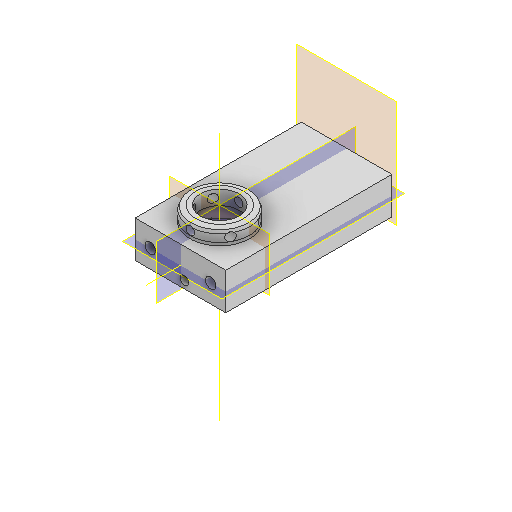
# Autodesk Inventor part: 30_Linear_Stage_NEMA11_arm_bayonetmount_femalemale
Saved by Autodesk Inventor 2022 (Build 260153000, 153)
## iProperties
Created: 2023-02-17
Part Number: 30_Linear_Stage_NEMA11_arm_bayonetmount_femalemale
Material: Generisch
Document SubType Name: Modeling
Designer: diederichbenedict
Density: 1 g/cm^3
Appearance: Vorgabe
Vendor: openUC2
Author: diederichbenedict
Autodesk Inventor part; units mm, degrees
ref_plane "YZ Plane" through (0, 0, 0) normal (1, 0, 0) x (0, 1, 0)
ref_plane "XZ Plane" through (0, 0, 0) normal (0, 1, 0) x (-1, 0, 0)
ref_plane "XY Plane" through (0, 0, 0) normal (0, 0, 1) x (1, 0, 0)
ref_plane "Arbeitsebene1" through (0, 0, 0) normal (0, 0, 1) x (1, 0, 0)
sketch "Skizze1" plane through (0, 0, 0) normal (0, 0, 1) x (1, 0, 0)
  line L0 (15, 26.050642) -> (15, 58.250642)
  line L1 (15, 58.250642) -> (-15, 58.250642)
  line L2 (-15, 58.250642) -> (-15, 26.050642)
  line L3 (-15, 26.050642) -> (15, 26.050642)
  circle A0 centre (10, 32.150642) radius 1.25
  circle A1 centre (-10, 32.150642) radius 1.25
  circle A2 centre (-10, 52.150642) radius 1.25
  circle A3 centre (10, 52.150642) radius 1.25
  circle A4 centre (7.5, 38.050642) radius 3.25
  circle A5 centre (7.5, 46.250642) radius 3.25
  circle A6 centre (-7.5, 38.050642) radius 3.25
  circle A7 centre (-7.5, 46.250642) radius 3.25
  line L4 (15, 26.050642) -> (-15, 26.050642)
  line L5 (-15, 26.050642) -> (-15, 42.150642)
  line L6 (-15, 42.150642) -> (15, 42.150642)
  line L7 (15, 42.150642) -> (15, 26.050642)
  circle A8 centre (10, 32.150642) radius 1.75
  circle A9 centre (-10, 32.150642) radius 1.75
  line L8 (-15, 38.250642) -> (15, 38.250642)
  point P0 (0, 0)
  dimension "d0" = 3.5
  dimension "d1" = 3.5
  dimension "d36" = 6.1
  constraints: 10 end point, 2 centre point, 2 coincident, 2 parallel, 2 perpendicular, 2 point on line, 1 horizontal, 1 midpoint
  measures "d0" diameter of A8
  measures "d1" diameter of A9
  measures "d36" distance from line of A1.centre L8
extrude "Extrusion1" add sketch "Skizze1" along normal blind 55 contours L3 L2 L8 A6 A4 L0 | A4 L8 | L8 A6 picked at (7.078886, 37.164115) picked at (-6.44731, 37.129778)
sketch "Skizze2" plane through (-15, 26.050642, 0) normal (0, -1, 0) x (1, 0, 0)
  circle A0 centre (15, -8) radius 4 projected
  circle A1 centre (15, 42) radius 10
  point P0 (15, 0)
  dimension "d4" = 20
  dimension "d5" = 50
  constraints: 1 centre point
  measures "d4" diameter of A1
  measures "d5" distance of A0.centre A1.centre
extrude "Extrusion2" cut sketch "Skizze2" against normal blind 60 contours A1
ref_plane "Arbeitsebene2" through (0, 26.050642, 0) normal (-1, 0, 0) x (0, 0, 1)
ref_plane "Arbeitsebene3" through (0, 26.050642, 42) normal (0, 0, 1) x (1, 0, 0)
sketch "Skizze3" plane through (0, 26.050642, 0) normal (-1, 0, 0) x (0, 0, 1)
  line L0 (32, 0) -> (32, 12.2)
  line L1 (32, 1.05) -> (30, 1.05)
  line L2 (30, 1.05) -> (30, 4.25)
  line L3 (30, 4.25) -> (32, 4.25)
  line L4 (32, 4.25) -> (32, 1.05)
  line L5 (0, 0) -> (55, 0)
  line L6 (25.530471, 4.35) -> (40.965559, 4.35)
  line L7 (25.530471, 4.35) -> (40.965559, 4.35) construction
  line L8 (42, 25.550128) -> (42, -34.65077)
  point P0 (0, -26.050642)
  dimension "d11" = 2
  dimension "d12" = 3.2
  dimension "d34" = 0
  dimension "d35" = 0.1
  dimension "d55" = 10
  constraints: 12 end point, 3 horizontal, 2 parallel, 1 collinear, 1 perpendicular, 1 point on line, 1 other
  measures "d11" distance of L2.end L3.end
  measures "d12" distance of L1.end L2.end
  measures "d34" distance between parallel lines of L6 L7
  measures "d35" distance from line of L6 L3.end
  measures "d55" distance between parallel lines of L0 L8
coil "Spirale1" sketch "Skizze3" operation cut axis through (0, 26.050642, 42) along (0, 1, 0) pitch 6 turns 0.15 hand right
sketch "Skizze4" plane through (0, 26.050642, 0) normal (-1, 0, 0) x (0, 0, 1)
  line L0 (32, 4.25) -> (30, 4.25)
  line L1 (30, 1.05) -> (32, 1.05)
  line L2 (32, 1.05) -> (30, 1.05)
  line L3 (30, 1.05) -> (30, -0.453392)
  line L4 (30, -0.453392) -> (32, -0.453392)
  line L5 (32, -0.453392) -> (32, 1.05)
  line L6 (32, 4.25) -> (30, 4.25)
  line L7 (30, 4.25) -> (30, -0.517938)
  line L8 (30, -0.517938) -> (32, -0.517938)
  line L9 (32, -0.517938) -> (32, 4.25)
  line L10 (42, -33.70077) -> (42, 19.850128)
  point P0 (0, -26.050642)
  constraints: 16 end point, 4 parallel, 2 horizontal, 2 perpendicular, 1 point on line
revolve "Umdrehung1" cut sketch "Skizze4" angle 20 about axis through (0, 26.050642, 42) along (0, -1, 0) contours L9 L1 L7 L0 | L5 L4 L3 L1
chamfer "Fase2" distance 0.5 angle 45 5 edges at (-7.0711, 26.0506, 49.0711) (8.1915, 26.0506, 36.2642) (3.7622, 26.0506, 31.6634) (0, 26.0506, 31) (2.0838, 26.0506, 30.1823)
chamfer "Fase3" distance 0.5 angle 45 1 edges at (0, 27.1006, 31)
ref_plane "Arbeitsebene4" through (-15, 32.150642, 0) normal (0, -1, 0) x (1, 0, 0)
pattern_circular "Runde Anordnung4" count 3 over 360 about axis through (0, 26.050642, 42) along (0, 1, 0) of "Umdrehung1", "Spirale1"
sketch "Skizze6" plane through (0, 26.050642, 0) normal (-1, 0, 0) x (0, 0, 1)
  spline S0 degree 3 poles (32.345316, 15.617608) (32.347206, 15.582897) (32.349028, 15.545933) (32.355973, 15.384441) (32.360157, 15.228443) (32.358854, 14.886362) (32.353087, 14.70028) (32.332312, 14.34843) (32.315768, 14.159486) (32.275946, 13.812033) (32.252953, 13.653484) (32.212647, 13.402974) (32.192672, 13.294176) (32.165012, 13.149587) (32.160563, 13.128127) (32.157596, 13.113821) (32.165012, 13.149587) (32.192672, 13.294176) (32.212647, 13.402974) (32.252953, 13.653484) (32.275946, 13.812033) (32.315768, 14.159486) (32.332312, 14.34843) (32.342785, 14.525804) (32.353087, 14.70028) (32.358854, 14.886362) (32.360157, 15.228443) (32.355973, 15.384441) (32.349028, 15.545933) (32.347206, 15.582897) (32.345316, 15.617608) knots -0.54731919 -0.54731919 -0.54731919 -0.54731919 -0.53094737 -0.53094737 -0.4785116 -0.4785116 -0.42607582 -0.42607582 -0.3727688 -0.3727688 -0.31946179 -0.31946179 -0.26624985 -0.26624985 -0.21303791 -0.21303791 -0.15982597 -0.15982597 -0.10661404 -0.10661404 -0.05330702 -0.05330702 0 0 0 0.05243578 0.05243578 0.10487155 0.10487155 0.12124336 0.12124336 0.12124336 0.12124336
  line L0 (0, 12.2) -> (55, 12.2)
  line L1 (32.103074, 12.2) -> (32.157596, 13.113821)
  line L2 (32.706285, 15.913821) -> (34.103074, 16.95)
  spline S1 degree 3 poles (32.345316, 15.617608) (32.360249, 15.629659) (32.374838, 15.641457) (32.477093, 15.724301) (32.560317, 15.792677) (32.675128, 15.887705) (32.693822, 15.903375) (32.706285, 15.913821) (32.675128, 15.887705) (32.560317, 15.792677) (32.477093, 15.724301) (32.374838, 15.641457) (32.360249, 15.629659) (32.345316, 15.617608) knots 0 0 0 0 0.0373764 0.0373764 0.2686882 0.2686882 0.5 0.5 0.7313118 0.7313118 0.9626236 0.9626236 1 1 1 1
  line L3 (49.896926, 16.95) -> (34.103074, 16.95)
  line L4 (35.603074, 16.95) -> (35.603074, 12.2)
  line L5 (51.958771, 11.9) -> (32.04123, 11.9)
  line L6 (32, 0.5) -> (32, 12.2)
  line L7 (35.603074, 12.2) -> (32, 6.10386)
  line L8 (32, 12.2) -> (32.103074, 12.2)
  line L9 (0, 12.2) -> (55, 12.2)
  line L10 (34.103074, 16.95) -> (32.514186, 16.551369)
  line L11 (32.514186, 16.551369) -> (32.345316, 15.617608)
  line L12 (34.103074, 16.95) -> (35.603074, 16.95)
  line L13 (42, 16.750684) -> (42, 2.215395)
  line L14 (32.157596, 13.113821) -> (32.157596, 15.617608)
  line L15 (32.157596, 15.617608) -> (32.514186, 16.551369)
  point P0 (0, -26.050642)
  constraints: 22 end point, 3 vertical, 2 collinear, 1 point on line, 8 other
revolve "Umdrehung2" add sketch "Skizze6" angle 360 about axis through (0, 42.801326, 42) along (0, -1, 0) contours L11 L10 L3 L4 L0 L1 L14 S0 | S0 L14 L15 L11 | L0 L7 L6
sketch "Skizze7" plane through (0, 26.050642, 42) normal (0, 0, 1) x (1, 0, 0)
  spline S0 degree 3 poles (-0.861194, 15.617608) (-0.905683, 15.582897) (-0.947481, 15.545933) (-1.1102, 15.384441) (-1.218098, 15.228443) (-1.362227, 14.886362) (-1.398455, 14.70028) (-1.401467, 14.34843) (-1.367345, 14.159486) (-1.225839, 13.812033) (-1.118475, 13.653484) (-0.870101, 13.402974) (-0.712517, 13.294176) (-0.36617, 13.149587) (-0.177373, 13.113821) (0.177373, 13.113821) (0.36617, 13.149587) (0.712517, 13.294176) (0.870101, 13.402974) (1.118475, 13.653484) (1.225839, 13.812033) (1.367345, 14.159486) (1.401467, 14.34843) (1.399949, 14.525804) (1.398455, 14.70028) (1.362227, 14.886362) (1.218098, 15.228443) (1.1102, 15.384441) (0.947481, 15.545933) (0.905683, 15.582897) (0.861194, 15.617608) knots -0.54731919 -0.54731919 -0.54731919 -0.54731919 -0.53094737 -0.53094737 -0.4785116 -0.4785116 -0.42607582 -0.42607582 -0.3727688 -0.3727688 -0.31946179 -0.31946179 -0.26624985 -0.26624985 -0.21303791 -0.21303791 -0.15982597 -0.15982597 -0.10661404 -0.10661404 -0.05330702 -0.05330702 0 0 0 0.05243578 0.05243578 0.10487155 0.10487155 0.12124336 0.12124336 0.12124336 0.12124336
  line L0 (0, 4.05) -> (0, 19.1)
  line L1 (19.6, 14.513821) -> (-19.6, 14.513821)
  circle A0 centre (0, 14.513821) radius 1.399997
  point P0 (0, -26.050642)
  constraints: 4 end point, 1 centre point, 1 horizontal, 1 midpoint, 1 vertical, 4 other
extrude "Extrusion4" cut sketch "Skizze7" along normal through all both and the other way through all
pattern_circular "Runde Anordnung5" count 6 over 360 about axis through (0, 40.416356, 42) along (0, 1, 0) of "Extrusion4"
sketch "Skizze8" plane through (0, 0, 55) normal (0, 0, 1) x (1, 0, 0)
  line L0 (-15, 38.250642) -> (-15, 26.050642)
  line L1 (-15, 26.050642) -> (15, 26.050642)
  line L2 (15, 26.050642) -> (15, 38.250642)
  line L3 (15, 38.250642) -> (-15, 38.250642)
  circle A0 centre (10, 32.150642) radius 1.75
  circle A1 centre (-10, 32.150642) radius 1.75
  circle A2 centre (1.266249, 28.522218) radius 1.4
  point P0 (0, 0)
  dimension "d56" = 2.8
  constraints: 1 centre point
  measures "d56" diameter of A2
extrude "Extrusion5" cut sketch "Skizze8" against normal blind 10 contours A2
